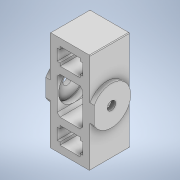
# Autodesk Inventor part: bottom idler housing
Saved by Autodesk Inventor 2020.4 (Build 244396000, 396)
## iProperties
Created: 2021-03-29
Part Number: bottom idler housing
Material: Generic
Document SubType Name: Modeling
Designer: AOB
Mass: 33.5422 g
Surface Area: 155.659 cm^2
Volume: 33.5422 cm^3
Density: 1 g/cm^3
Appearance: Default
Author: AOB
Autodesk Inventor part; units mm, degrees
ref_plane "YZ Plane" through (0, 0, 0) normal (1, 0, 0) x (0, 1, 0)
ref_plane "XZ Plane" through (0, 0, 0) normal (0, 1, 0) x (-1, 0, 0)
ref_plane "XY Plane" through (0, 0, 0) normal (0, 0, 1) x (1, 0, 0)
sketch "Sketch1" plane through (0, 0, 0) normal (0, 0, 1) x (1, 0, 0)
  line L0 (0, 0) -> (28, 0)
  line L1 (28, 0) -> (28, -70)
  line L2 (28, -70) -> (0, -70)
  line L3 (0, -70) -> (0, 0)
  line L4 (7, -22) -> (21, -22)
  line L5 (23, -24) -> (23, -46)
  line L6 (21, -48) -> (7, -48)
  line L7 (5, -46) -> (5, -24)
  line L8 (7, -53) -> (21, -53)
  line L9 (23, -55) -> (23, -63)
  line L10 (21, -65) -> (7, -65)
  line L11 (5, -63) -> (5, -55)
  line L12 (7, -5) -> (21, -5)
  line L13 (23, -7) -> (23, -15)
  line L14 (21, -17) -> (7, -17)
  line L15 (5, -15) -> (5, -7)
  line L16 (23, -7) -> (21, -7)
  line L17 (21, -7) -> (21, -5)
  line L18 (7, -7) -> (5, -7)
  line L19 (23, -63) -> (21, -63)
  line L20 (21, -63) -> (21, -65)
  line L21 (7, -65) -> (7, -63)
  line L22 (5, -63) -> (7, -63)
  line L23 (21, -53) -> (21, -55)
  line L24 (21, -55) -> (23, -55)
  line L25 (7, -53) -> (7, -55)
  line L26 (7, -55) -> (5, -55)
  line L27 (21, -48) -> (23, -46)
  line L28 (5, -46) -> (7, -48)
  line L29 (23, -24) -> (21, -22)
  line L30 (5, -24) -> (7, -22)
  line L31 (23, -15) -> (21, -15)
  line L32 (21, -15) -> (21, -17)
  line L33 (7, -17) -> (7, -15)
  line L34 (7, -15) -> (5, -15)
  line L35 (7, -7) -> (7, -5)
  point P0 (23, -48)
  point P1 (5, -48)
  point P2 (23, -22)
  point P3 (5, -22)
  dimension "d1" = 28
  dimension "d4" = 5
  dimension "d7" = 5
  dimension "d8" = 5
  dimension "d10" = 22
  dimension "d50" = 22
  dimension "d59" = 2
  dimension "d62" = 2
  dimension "d67" = 5
  dimension "d68" = 5
  constraints: 72 end point, 13 point on line, 12 perpendicular, 9 parallel, 5 horizontal, 2 vertical
  measures "d1" distance of L0.start L0.end
  measures "d4" distance between parallel lines of L1 L5
  measures "d7" distance between parallel lines of L2 L10
  measures "d8" distance between parallel lines of L6 L8
  measures "d10" distance between parallel lines of L0 L4
  measures "d50" distance between parallel lines of L2 L6
  measures "d59" distance of L6.start point (23, -48)
  measures "d62" distance of L6.end point (5, -48)
  measures "d67" distance between parallel lines of L4 L14
  measures "d68" distance between parallel lines of L0 L12
extrude "Extrusion1" add sketch "Sketch1" against normal blind 24
sketch "Sketch2" plane through (0, 0, -24) normal (0, 0, -1) x (1, 0, 0)
  line L0 (0, 0) -> (28, 0) projected
  line L1 (0, 70) -> (0, 0) projected
  line L2 (28, 0) -> (28, 70) projected
  line L3 (28, 70) -> (0, 70) projected
extrude "Extrusion2" add sketch "Sketch2" along normal blind 4
sketch "Sketch3" plane through (23, -42, 0) normal (-1, 0, 0) x (0, 0, -1)
  line L0 (0, -18) -> (0, 4) projected
  line L1 (0, 4) -> (24, 4) projected
  line L2 (24, 4) -> (24, -18) projected
  line L3 (0, -18) -> (24, -18) projected
  line L4 (0, 4) -> (24, 4) projected
  line L5 (0, -18) -> (24, -18) projected
  line L6 (24, 4) -> (12, -7)
  line L7 (0, 4) -> (12, -7)
  point P0 (1, 7)
  constraints: 4 end point
fillet "Fillet1" radius 0.5 1 edges at (28, 0, -14)
fillet "Fillet2" radius 0.5 8 edges at (27.8536, -0.1464, -28) (28, -35.25, -28) (13.75, 0, -28) (0, -35, -28) (0, 0, -14) (0, -70, -14) (14, -70, -28) (28, -70, -14)
hole "Hole1" at (23, -35, -12) direction (1, 0, 0) diameter 22 end through all both
sketch "Sketch8" plane through (0, -69.5, 0) normal (-1, 0, 0) x (0, 0, 1)
  circle A0 centre (-12, 34.5) radius 11 projected
  circle A1 centre (-12, 34.5) radius 11.5
  point P0 (0, 69.5)
  dimension "d95" = 23
  constraints: 1 centre point, 1 coincident
  measures "d95" diameter of A1
extrude "Extrusion3" cut sketch "Sketch8" against normal blind 1
sketch "Sketch7" plane through (0, -69.5, 0) normal (-1, 0, 0) x (0, 0, 1)
  arc A0 (0, 40.6847) -> (0, 28.3153) centre (-12, 34.5) ccw
  circle A1 centre (-12, 34.5) radius 3
  line L0 (0, 40.6847) -> (0, 28.3153)
  line L1 (0, 0) -> (0, 69)
  point P0 (0, 69.5)
  constraints: 4 end point, 2 centre point, 2 point on circle
extrude "Extrusion4" add sketch "Sketch7" along normal blind 3
ref_plane "Work Plane1" through (14, -69.5, -27.5) normal (-1, 0, 0) x (0, 0, 1)
mirror "Mirror1" about plane through (14, -69.5, -27.5) normal (-1, 0, 0) of "Extrusion4", "Extrusion3"
equation "\"d62\" = d61"
equation "\"d61\" = d59"
body "Solid1"
